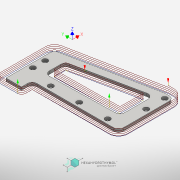
# Autodesk Inventor part: C-head-side
Saved by Autodesk Inventor 2016 (Build 200138000, 138)
## iProperties
Created: 2015-05-08
Part Number: C-head-side
Material: Generic
Document SubType Name: Modeling
Designer: ax
Density: 1 g/cm^3
Appearance: Default
Mass: 2.37553 g
Surface Area: 31.8271 cm^2
Volume: 2.37553 cm^3
Author: ax
Autodesk Inventor part; units mm, degrees
ref_plane "YZ Plane" through (0, 0, 0) normal (1, 0, 0) x (0, 1, 0)
ref_plane "XZ Plane" through (0, 0, 0) normal (0, 1, 0) x (-1, 0, 0)
ref_plane "XY Plane" through (0, 0, 0) normal (0, 0, 1) x (1, 0, 0)
sketch "Sketch1" plane through (0, 0, 0) normal (0, 0, 1) x (1, 0, 0)
  line L0 (0, 0) -> (0, 36)
  line L1 (0, 36) -> (66, 36)
  line L2 (66, 36) -> (66, -7)
  line L3 (66, -7) -> (0, -7)
  line L4 (0, -7) -> (0, 0)
  dimension "d24" = 36
  dimension "d26" = 66
  dimension "d27" = 43
  dimension "d28" = 66
  constraints: 10 end point, 2 perpendicular, 1 point on line, 1 vertical
  measures "d24" distance of L0.start L0.end
  measures "d26" distance of L0.end L1.end
  measures "d27" distance of L1.end L2.end
  measures "d28" distance of L2.end L3.end
extrude "Extrusion1" add sketch "Sketch1" along normal blind 2
sketch "Sketch2" plane through (0, 0, 2) normal (0, 0, 1) x (1, 0, 0)
  line L0 (0, 36) -> (66, 36) projected
  line L1 (0, 36) -> (60, 36)
  line L2 (0, 36) -> (0, -7) projected
  line L3 (0, 36) -> (0, 24)
  line L4 (0, -7) -> (66, -7) projected
  line L5 (0, 24) -> (60, 36)
  line L6 (11, -7) -> (11, 0)
  point P0 (0, 0)
  dimension "d29" = 60
  dimension "d31" = 12
  dimension "d60" = 43
  constraints: 8 end point, 3 point on line, 1 vertical
  measures "d29" distance of L0.start L1.end
  measures "d31" distance of L0.start L3.end
  measures "d60" distance between parallel lines of L4 L0
extrude "Extrusion2" cut sketch "Sketch2" against normal through all
sketch "Sketch3" plane through (0, 0, 2) normal (0, 0, 1) x (1, 0, 0)
  point P0 (63, 21)
  point P1 (63, 33)
hole "Hole1" at (63, 21, 2) at (63, 33, 2) direction (0, 0, -1) diameter 3.4 depth 2
sketch "Sketch4" plane through (0, 0, 2) normal (0, 0, 1) x (1, 0, 0)
  point P0 (19, 3)
  point P1 (37.5, 3)
  point P2 (56, 3)
hole "Hole3" at (19, 3, 2) at (37.5, 3, 2) at (56, 3, 2) direction (0, 0, -1) diameter 3.4 depth 2
sketch "Sketch5" plane through (0, 0, 0) normal (0, 0, -1) x (-1, 0, 0)
  point P0 (-3, 15.4)
  point P1 (-3, 7.4)
hole "Hole5" at (3, 15.4, 0) at (3, 7.4, 0) direction (0, 0, 1) diameter 3.4 depth 2
sketch "Sketch6" plane through (0, 0, 2) normal (0, 0, 1) x (1, 0, 0)
  line L0 (66, -7) -> (10, -7)
  line L1 (10, -7) -> (10, 0)
  line L2 (10, 0) -> (66, 0)
  line L3 (66, 0) -> (66, -7)
  point P0 (0, 0)
  constraints: 8 end point, 2 parallel, 1 horizontal, 1 perpendicular
extrude "Extrusion3" cut sketch "Sketch6" against normal through all
sketch "Sketch7" plane through (0, 0, 2) normal (0, 0, 1) x (1, 0, 0)
  line L0 (13.1646, 8.0659) -> (54.9646, 8.9368)
  line L1 (58, 12.0361) -> (58, 27.1876)
  line L2 (54.2677, 30.2224) -> (12.4677, 21.5141)
  line L3 (10, 18.4793) -> (10, 11.1653)
  arc A0 (54.9646, 8.9368) -> (58, 12.0361) centre (54.9, 12.0361) ccw
  arc A1 (58, 27.1876) -> (54.2677, 30.2224) centre (54.9, 27.1876) ccw
  arc A2 (12.4677, 21.5141) -> (10, 18.4793) centre (13.1, 18.4793) ccw
  arc A3 (10, 11.1653) -> (13.1646, 8.0659) centre (13.1, 11.1653) ccw
  point P0 (0, 0)
  dimension "d63" = 3.1
  constraints: 8 end point, 8 point on circle, 8 tangent, 4 centre point, 3 equal radius, 1 parallel, 1 vertical
  measures "d63" radius of A0
extrude "Extrusion4" cut sketch "Sketch7" against normal through all
fillet "Fillet1" radius 3.1 5 edges at (66, 0, 1) (10, 0, 1) (0, 24, 1) (60, 36, 1) (66, 36, 1)
equation "\"d24\" = d2 + cMotorSize"
equation "\"d26\" = d0"
equation "\"d28\" = d0"
equation "\"d0\" = 66"
equation "\"d2\" = 6"
equation "\"cMotorSize\" = 30"
body "Solid1"
